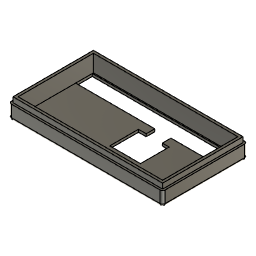
Caixa Sensores - Base (Autodesk Fusion 360 design; units mm, degrees)
Autodesk Fusion 360 part; units mm, degrees
sketch "Esboço1" plane through (0, 0, 0) normal (0, 0, 1) x (1, 0, 0)
  line L0 (30, -16.5) -> (-30, -16.5)
  line L1 (-30, -16.5) -> (-30, 16.5)
  line L2 (-30, 16.5) -> (30, 16.5)
  line L3 (30, 16.5) -> (30, -16.5)
  line L4 (30, -16.5) -> (-30, 16.5) construction
  line L5 (-30, -16.5) -> (30, 16.5) construction
  dimension "d1" = 60
  dimension "d2" = 33
  constraint horizontal L0
  constraint perpendicular L0 L1
  constraint parallel L0 L2
  constraint parallel L1 L3
  constraint coincident L4 origin
  constraint coincident L5 origin
  measures "d1" distance of L1.end L2.end
  measures "d2" distance of L0.end L1.end
extrude "Extrusão1" add sketch "Esboço1" along normal blind 7
shell "Casca1" thickness 1.4 removed faces 1 at (-10, -5.5, 7)
sketch "Esboço2" plane through (0, 0, 1.4) normal (0, 0, 1) x (-1, 0, 0)
  line L0 (-28.6, -15.1) -> (28.6, -15.1)
  line L1 (28.6, -15.1) -> (28.6, 15.1)
  line L2 (28.6, 15.1) -> (-28.6, 15.1)
  line L3 (-28.6, 15.1) -> (-28.6, -15.1)
  line L4 (-28.3059, -7.7483) -> (28.1941, -7.7483)
  line L5 (28.1941, -7.7483) -> (28.1941, -14.2483)
  line L6 (28.1941, -14.2483) -> (-28.3059, -14.2483)
  line L7 (-28.3059, -14.2483) -> (-28.3059, -7.7483)
  line L8 (-28.3059, -7.7483) -> (28.1941, -14.2483) construction
  line L9 (28.1941, -7.7483) -> (-28.3059, -14.2483) construction
  point P0 (-0.0559, -10.9983)
  dimension "d6" = 56.5
  dimension "d7" = 6.5
  constraint horizontal L4
  constraint perpendicular L4 L5
  constraint parallel L4 L6
  constraint parallel L5 L7
  constraint coincident L8 P0
  constraint coincident L9 P0
  measures "d6" distance of L5.end L6.end
  measures "d7" distance of L4.end L5.end
extrude "Extrusão2" cut sketch "Esboço2" against normal blind 1 contours L0 L1 L2 L3 | L4 L5 L6 L7
sketch "Esboço3" plane through (0, 0, 0.4) normal (0, 0, 1) x (-1, 0, 0)
  line L0 (-27.375, -7.75) -> (27.375, -7.75)
  line L1 (27.375, -7.75) -> (27.375, 16.1)
  line L2 (27.375, 16.1) -> (-27.375, 16.1)
  line L3 (-27.375, 16.1) -> (-27.375, -7.75)
  line L4 (0, 3) -> (0.325, 3)
  line L5 (0.325, 3) -> (0.325, 6.8)
  line L6 (0.325, 6.8) -> (-11.675, 6.8)
  line L7 (-11.675, 6.8) -> (-11.675, 3)
  line L8 (0.325, 3) -> (0.325, -4.4)
  line L9 (0.325, -4.4) -> (-11.675, -4.4)
  line L10 (-11.675, -4.4) -> (-11.675, 6.8)
  line L11 (0.325, -4.4) -> (0.325, -7.75)
  line L12 (-2.7067, -7.75) -> (-2.7067, -4.4)
  line L13 (-2.7067, -7.75) -> (0.325, -7.75)
  line L14 (-11.675, -4.4) -> (-11.675, -7.75)
  line L15 (-8.9983, -7.75) -> (-8.9983, -4.4)
  line L16 (-8.9983, -7.75) -> (-11.675, -7.75)
  dimension "d24" = 3.8
  dimension "d25" = 7.4
  constraint perpendicular L4 L5
  constraint perpendicular L4 L8
  constraint perpendicular L6 L10
  constraint coincident L0 L11.end
  constraint perpendicular L0 L11
  constraint coincident L0 L12.start
  constraint coincident L9 L12.end
  constraint perpendicular L9 L12
  constraint coincident L0 L14.end
  constraint perpendicular L0 L14
  constraint coincident L0 L15.start
  constraint coincident L9 L15.end
  constraint perpendicular L9 L15
  measures "d24" distance of L4.end L5.end
  measures "d25" distance of L4.end L8.end
extrude "Extrusão8" cut sketch "Esboço3" against normal blind 1 contours L0 L9 L12 L15
extrude "Extrusão6" cut sketch "Esboço3" against normal blind 1 contours L5 L6 L7 L8 L9 L10
extrude "Extrusão5" cut sketch "Esboço2" against normal blind 2 contours L4 L5 L6 L7
move_face "Faces de deslocamento1" offset 0.4 4 faces at (-28.6, 5.0333, 2.6) (9.5333, 15.1, 4.8) (-9.5333, -15.1, 4.8) (28.6, 5.0333, 4.8)
sketch "Esboço4" plane through (0, 0, 7) normal (0, 0, 1) x (-1, 0, 0)
  line L0 (-28.2, -14.7) -> (-28.2, 14.7)
  line L1 (-28.2, 14.7) -> (28.2, 14.7)
  line L2 (28.2, 14.7) -> (28.2, -14.7)
  line L3 (28.2, -14.7) -> (-28.2, -14.7)
  line L4 (-30, -16.5) -> (30, -16.5)
  line L5 (30, -16.5) -> (30, 16.5)
  line L6 (30, 16.5) -> (-30, 16.5)
  line L7 (-30, 16.5) -> (-30, -16.5)
  line L8 (-29.2, 15.7) -> (29.2, 15.7)
  line L9 (29.2, 15.7) -> (29.2, -15.7)
  line L10 (29.2, -15.7) -> (-29.2, -15.7)
  line L11 (-29.2, -15.7) -> (-29.2, 15.7)
  line L12 (-29.2, 15.7) -> (29.2, -15.7) construction
  line L13 (29.2, 15.7) -> (-29.2, -15.7) construction
  dimension "d17" = 58.4
  dimension "d18" = 31.4
  constraint horizontal L8
  constraint perpendicular L8 L9
  constraint parallel L8 L10
  constraint parallel L9 L11
  constraint coincident L12 origin
  constraint coincident L13 origin
  measures "d17" distance of L9.end L10.end
  measures "d18" distance of L8.end L9.end
extrude "Extrusão4" cut sketch "Esboço4" against normal blind 2 contours L4 L5 L6 L7
move_face "Faces de deslocamento2" offset 0.6 1 faces at (-19.5064, -5.1839, 0)
fillet "Arredondamento1" radius 1 4 edges at (30, -16.5, 2.2) (30, 16.5, 2.2) (-30, 16.5, 2.2) (-30, -16.5, 2.2)
fillet "Arredondamento2" radius 1 8 edges at (30, 0, -0.6) (29.7071, 16.2071, -0.6) (0, 16.5, -0.6) (-29.7071, 16.2071, -0.6) (-30, 0, -0.6) (-29.7071, -16.2071, -0.6) (0, -16.5, -0.6) (29.7071, -16.2071, -0.6)
